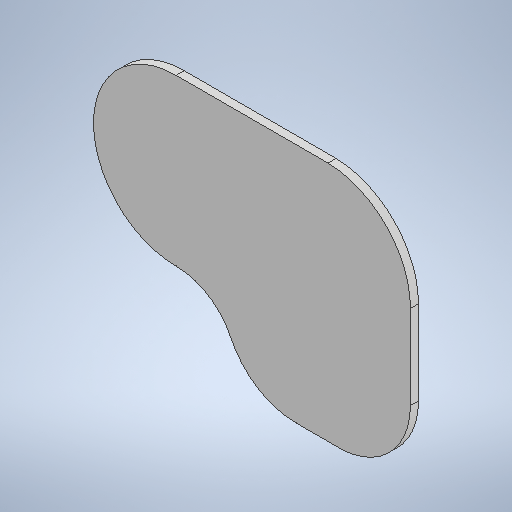
# Autodesk Inventor part: Peça2
Saved by Autodesk Inventor 2025.2 (Build 292293000, 293)
## iProperties
Created: 2025-06-03
Part Number: Peça2
Material: Genérico
Document SubType Name: Modeling
Designer: Gustavo Sousa
Density: 1 g/cm^3
Appearance: Padrão
Author: Gustavo Sousa
Autodesk Inventor part; units mm, degrees
sketch "Esboço1" plane through (0, 0, 0) normal (0, 0, 1) x (1, 0, 0)
  arc A0 (0, 20.5) -> (0, -20.5) centre (0, 0) ccw
  line L0 (0, 20.5) -> (37.722, 20.5)
  arc A1 (58.146, -0.535) -> (37.722, 20.5) centre (37.146, -0.4921) ccw
  line L1 (58.146, -0.535) -> (58.146, -21.396)
  arc A2 (41.6369, -39.3342) -> (58.146, -21.396) centre (40.146, -21.396) ccw
  line L2 (29.8049, -39.3342) -> (41.6369, -39.3342)
  arc A3 (13.5477, -29.061) -> (0, -20.5) centre (0, -35.5) ccw
  arc A4 (13.5477, -29.061) -> (29.8049, -39.3342) centre (29.8049, -21.3342) ccw
  dimension "d6" = 20.5
  dimension "d7" = 37.722
  dimension "d8" = 21
  dimension "d10" = 20.861
  dimension "d11" = 58.146
  dimension "d13" = 37.146
  dimension "d14" = 18
  dimension "d16" = 11.832
  dimension "d18" = 15
  dimension "d19" = 35.5
  dimension "d23" = 18
  constraints: 10 point on circle, 6 end point, 5 centre point, 3 tangent, 2 horizontal, 2 vertical alignment, 1 coincident, 1 vertical
  measures "d6" radius of A0
  measures "d7" distance of L0.start L0.end
  measures "d8" radius of A1
  measures "d10" distance of L1.start L1.end
  measures "d11" horizontal distance of L1.start point (0, 0)
  measures "d13" horizontal distance of point (0, 0) A1.centre
  measures "d14" radius of A2
  measures "d16" distance of L2.start L2.end
  measures "d18" radius of A3
  measures "d19" distance of A0.centre A3.centre
  measures "d23" radius of A4
extrude "Extrusão1" add sketch "Esboço1" along normal mid plane 2
